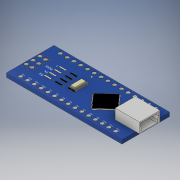
# Autodesk Inventor part: Arduino Nano
Saved by Autodesk Inventor 2019 (Build 230136000, 136)
## iProperties
Created: 2019-04-20
Part Number: Arduino Nano
Material: Generic
Document SubType Name: Modeling
Designer: richc
Density: 1 g/cm^3
Appearance: Default
Author: richc
Autodesk Inventor part; units mm, degrees
ref_plane "YZ Plane" through (0, 0, 0) normal (1, 0, 0) x (0, 1, 0)
ref_plane "XZ Plane" through (0, 0, 0) normal (0, 1, 0) x (-1, 0, 0)
ref_plane "XY Plane" through (0, 0, 0) normal (0, 0, 1) x (1, 0, 0)
sketch "Sketch1" plane through (0, 0, 0) normal (0, 1, 0) x (-1, 0, 0)
  line L0 (17.3155, -3.1926) -> (-25.8645, -3.1926)
  line L1 (-25.8645, -3.1926) -> (-25.8645, 14.5874)
  line L2 (-25.8645, 14.5874) -> (17.3155, 14.5874)
  line L3 (17.3155, 14.5874) -> (17.3155, -3.1926)
  point P0 (0, 0)
  dimension "d0" = 43.18
  dimension "d1" = 17.78
  constraints: 8 end point, 2 parallel, 1 horizontal, 1 perpendicular
  measures "d0" distance of L1.end L2.end
  measures "d1" distance of L0.end L1.end
extrude "Extrusion1" add sketch "Sketch1" along normal blind 1.524
sketch "Sketch2" plane through (0, 1.524, 0) normal (0, 1, 0) x (1, 0, 0)
  circle A0 centre (-13.5055, -13.1177) radius 0.635
  line L0 (25.8645, 3.1926) -> (-17.3155, 3.1926) projected
  line L1 (-17.3155, 3.1926) -> (-17.3155, -14.5874) projected
  line L2 (-17.3155, -14.5874) -> (25.8645, -14.5874) projected
  line L3 (25.8645, -14.5874) -> (25.8645, 3.1926) projected
  circle A1 centre (-10.9655, -13.1177) radius 0.635
  circle A2 centre (-8.4255, -13.1177) radius 0.635
  circle A3 centre (-5.8855, -13.1177) radius 0.635
  circle A4 centre (-3.3455, -13.1177) radius 0.635
  circle A5 centre (-0.8055, -13.1177) radius 0.635
  circle A6 centre (1.7345, -13.1177) radius 0.635
  circle A7 centre (4.2745, -13.1177) radius 0.635
  circle A8 centre (6.8145, -13.1177) radius 0.635
  circle A9 centre (9.3545, -13.1177) radius 0.635
  circle A10 centre (11.8945, -13.1177) radius 0.635
  circle A11 centre (14.4345, -13.1177) radius 0.635
  circle A12 centre (16.9745, -13.1177) radius 0.635
  circle A13 centre (19.5145, -13.1177) radius 0.635
  circle A14 centre (22.0545, -13.1177) radius 0.635
  line L4 (-17.3155, -5.6974) -> (-10.9655, -5.6974)
  circle A15 centre (-13.5055, 1.7229) radius 0.635
  line L5 (-17.3155, 3.1926) -> (25.8645, 3.1926)
  circle A16 centre (-10.9655, 1.7229) radius 0.635
  circle A17 centre (-8.4255, 1.7229) radius 0.635
  circle A18 centre (-5.8855, 1.7229) radius 0.635
  circle A19 centre (-3.3455, 1.7229) radius 0.635
  circle A20 centre (-0.8055, 1.7229) radius 0.635
  circle A21 centre (1.7345, 1.7229) radius 0.635
  circle A22 centre (4.2745, 1.7229) radius 0.635
  circle A23 centre (6.8145, 1.7229) radius 0.635
  circle A24 centre (9.3545, 1.7229) radius 0.635
  circle A25 centre (11.8945, 1.7229) radius 0.635
  circle A26 centre (14.4345, 1.7229) radius 0.635
  circle A27 centre (16.9745, 1.7229) radius 0.635
  circle A28 centre (19.5145, 1.7229) radius 0.635
  circle A29 centre (22.0545, 1.7229) radius 0.635
  point P0 (0, 0)
  dimension "d4" = 1.27
  dimension "d7" = 2.54
  dimension "d12" = 3.81
  constraints: 30 centre point, 15 symmetric about line, 4 end point, 2 horizontal, 1 midpoint, 43 other
  measures "d4" diameter of A0
  measures "d7" distance of A0.centre A1.centre
  measures "d12" distance from line of L1 A0.centre
extrude "Extrusion2" cut sketch "Sketch2" against normal blind 25.4 contours A0 | A1 | A2 | A3 | A4 | A5 | A6 | A7 | A8 | A9 | A10 | A11 | A12 | A13 | A14 | A15 | A16 | A17 | A18 | A19 | A20 | A21 | A22 | A23 | A24 | A25 | A26 | A27 | A28 | A29
sketch "Sketch3" plane through (0, 1.524, 0) normal (0, 1, 0) x (1, 0, 0)
  line L0 (25.8645, 3.1926) -> (-17.3155, 3.1926) projected
  line L1 (-17.3155, -14.5874) -> (25.8645, -14.5874) projected
  line L2 (10.4238, -10.3015) -> (15.5314, -5.7251)
  line L3 (15.5314, -5.7251) -> (10.9549, -0.6174)
  line L4 (5.8473, -5.1939) -> (10.9549, -0.6174)
  line L5 (5.8473, -5.1939) -> (10.4238, -10.3015)
  point P0 (0, 0)
  dimension "d26" = 6.858
  dimension "d27" = 6.858
  dimension "d28" = 6.858
  dimension "d29" = 6.858
  dimension "d75" = 90
  dimension "d76" = 3.81
  dimension "d77" = 4.2859
  constraints: 8 end point, 1 coincident
  measures "d26" distance of L4.start L2.start
  measures "d27" distance of L4.start L3.end
  measures "d28" distance of L2.end L3.end
  measures "d29" distance of L2.start L2.end
  measures "d75" angle of L2 L3
  measures "d76" distance from line of L0 L3.end
  measures "d77" distance from line of L1 L2.start
extrude "Extrusion3" add sketch "Sketch3" along normal blind 0.254
sketch "Sketch4" plane through (0, 1.524, 0) normal (0, 1, 0) x (1, 0, 0)
  circle A0 centre (-13.5055, 1.7229) radius 0.635 projected
  circle A1 centre (-13.5055, 1.7229) radius 0.7366
  line L0 (10.4238, -10.3015) -> (5.8473, -5.1939) projected
  line L1 (5.8473, -5.1939) -> (10.9549, -0.6174) projected
  line L2 (10.9549, -0.6174) -> (15.5314, -5.7251) projected
  line L3 (15.5314, -5.7251) -> (10.4238, -10.3015) projected
  circle A2 centre (-10.9655, 1.7229) radius 0.635 projected
  circle A3 centre (-5.8855, 1.7229) radius 0.635 projected
  circle A4 centre (1.7345, 1.7229) radius 0.635 projected
  circle A5 centre (22.0545, 1.7229) radius 0.635 projected
  circle A6 centre (14.4345, 1.7229) radius 0.635 projected
  circle A7 centre (9.3545, 1.7229) radius 0.635 projected
  circle A8 centre (4.2745, 1.7229) radius 0.635 projected
  circle A9 centre (22.0545, -13.1177) radius 0.635 projected
  circle A10 centre (16.9745, -13.1177) radius 0.635 projected
  circle A11 centre (11.8945, -13.1177) radius 0.635 projected
  circle A12 centre (6.8145, -13.1177) radius 0.635 projected
  circle A13 centre (1.7345, -13.1177) radius 0.635 projected
  circle A14 centre (-3.3455, -13.1177) radius 0.635 projected
  circle A15 centre (-8.4255, -13.1177) radius 0.635 projected
  circle A16 centre (-13.5055, -13.1177) radius 0.635 projected
  circle A17 centre (-10.9655, -13.1177) radius 0.635 projected
  circle A18 centre (-5.8855, -13.1177) radius 0.635 projected
  circle A19 centre (-0.8055, -13.1177) radius 0.635 projected
  circle A20 centre (4.2745, -13.1177) radius 0.635 projected
  circle A21 centre (9.3545, -13.1177) radius 0.635 projected
  circle A22 centre (14.4345, -13.1177) radius 0.635 projected
  circle A23 centre (19.5145, -13.1177) radius 0.635 projected
  circle A24 centre (-13.5055, 1.7229) radius 0.635 projected
  circle A25 centre (6.8145, 1.7229) radius 0.635 projected
  circle A26 centre (11.8945, 1.7229) radius 0.635 projected
  circle A27 centre (16.9745, 1.7229) radius 0.635 projected
  circle A28 centre (19.5145, 1.7229) radius 0.635 projected
  circle A29 centre (-3.3455, 1.7229) radius 0.635 projected
  circle A30 centre (-8.4255, 1.7229) radius 0.635 projected
  circle A31 centre (-0.8055, 1.7229) radius 0.635 projected
  line L4 (25.8645, 3.1926) -> (-17.3155, 3.1926) projected
  line L5 (-17.3155, 3.1926) -> (-17.3155, -14.5874) projected
  line L6 (-17.3155, -14.5874) -> (25.8645, -14.5874) projected
  line L7 (25.8645, -14.5874) -> (25.8645, 3.1926) projected
  circle A32 centre (-10.9655, 1.7229) radius 0.7366
  circle A33 centre (-8.4255, 1.7229) radius 0.7366
  circle A34 centre (-5.8855, 1.7229) radius 0.7366
  circle A35 centre (-3.3455, 1.7229) radius 0.7366
  circle A36 centre (-0.8055, 1.7229) radius 0.7366
  circle A37 centre (1.7345, 1.7229) radius 0.7366
  circle A38 centre (4.2745, 1.7229) radius 0.7366
  circle A39 centre (6.8145, 1.7229) radius 0.7366
  circle A40 centre (9.3545, 1.7229) radius 0.7366
  circle A41 centre (11.8945, 1.7229) radius 0.7366
  circle A42 centre (14.4345, 1.7229) radius 0.7366
  circle A43 centre (16.9745, 1.7229) radius 0.7366
  circle A44 centre (19.5145, 1.7229) radius 0.7366
  circle A45 centre (22.0545, 1.7229) radius 0.7366
  line L8 (-17.3155, 3.1926) -> (-17.3155, -14.5874) projected
  line L9 (-17.3155, -5.6974) -> (-11.7939, -5.6974)
  circle A46 centre (-13.5055, -13.1177) radius 0.635
  circle A47 centre (-13.5055, -13.1177) radius 0.7366
  circle A48 centre (-10.9655, -13.1177) radius 0.635
  circle A49 centre (-5.8855, -13.1177) radius 0.635
  circle A50 centre (1.7345, -13.1177) radius 0.635
  circle A51 centre (22.0545, -13.1177) radius 0.635
  circle A52 centre (14.4345, -13.1177) radius 0.635
  circle A53 centre (9.3545, -13.1177) radius 0.635
  circle A54 centre (4.2745, -13.1177) radius 0.635
  circle A55 centre (-13.5055, -13.1177) radius 0.635
  circle A56 centre (6.8145, -13.1177) radius 0.635
  circle A57 centre (11.8945, -13.1177) radius 0.635
  circle A58 centre (16.9745, -13.1177) radius 0.635
  circle A59 centre (19.5145, -13.1177) radius 0.635
  circle A60 centre (-3.3455, -13.1177) radius 0.635
  circle A61 centre (-8.4255, -13.1177) radius 0.635
  circle A62 centre (-0.8055, -13.1177) radius 0.635
  line L10 (25.8645, -14.5874) -> (-17.3155, -14.5874)
  line L11 (-17.3155, -14.5874) -> (-17.3155, 3.1926)
  line L12 (25.8645, 3.1926) -> (25.8645, -14.5874)
  circle A63 centre (-10.9655, -13.1177) radius 0.7366
  circle A64 centre (-8.4255, -13.1177) radius 0.7366
  circle A65 centre (-5.8855, -13.1177) radius 0.7366
  circle A66 centre (-3.3455, -13.1177) radius 0.7366
  circle A67 centre (-0.8055, -13.1177) radius 0.7366
  circle A68 centre (1.7345, -13.1177) radius 0.7366
  circle A69 centre (4.2745, -13.1177) radius 0.7366
  circle A70 centre (6.8145, -13.1177) radius 0.7366
  circle A71 centre (9.3545, -13.1177) radius 0.7366
  circle A72 centre (11.8945, -13.1177) radius 0.7366
  circle A73 centre (14.4345, -13.1177) radius 0.7366
  circle A74 centre (16.9745, -13.1177) radius 0.7366
  circle A75 centre (19.5145, -13.1177) radius 0.7366
  circle A76 centre (22.0545, -13.1177) radius 0.7366
  line L13 (-17.3155, -14.5874) -> (-17.3155, 3.1926)
  point P0 (0, 0)
  point P1 (0, -11.3949)
  dimension "d30" = 1.4732
  dimension "d33" = 2.54
  constraints: 46 centre point, 36 symmetric about line, 10 end point, 2 coincident, 2 horizontal, 1 midpoint, 59 other
  measures "d30" diameter of A1
  measures "d33" distance of A1.centre A32.centre
extrude "Extrusion4" add sketch "Sketch4" along normal blind 0.0025 contours A1 | A32 | A33 | A34 | A35 | A36 | A37 | A38 | A39 | A40 | A41 | A42 | A43 | A44 | A45 | A47 | A63 | A64 | A65 | A66 | A67 | A68 | A69 | A70 | A71 | A72 | A73 | A74 | A75 | A76
sketch "Sketch9" plane through (0, 1.524, 0) normal (0, 1, 0) x (1, 0, 0)
  line L0 (18.2445, -1.8874) -> (27.3885, -1.8874)
  line L1 (27.3885, -1.8874) -> (27.3885, -9.5074)
  line L2 (27.3885, -9.5074) -> (18.2445, -9.5074)
  line L3 (18.2445, -9.5074) -> (18.2445, -1.8874)
  line L4 (25.8645, -14.5874) -> (25.8645, 3.1926) projected
  line L5 (25.8645, -5.6974) -> (20.0043, -5.6974)
  point P0 (0, 0)
  dimension "d91" = 9.144
  dimension "d92" = 7.62
  dimension "d93" = 1.524
  constraints: 10 end point, 2 horizontal, 2 parallel, 1 midpoint, 1 perpendicular, 1 other
  measures "d91" distance of L1.end L2.end
  measures "d92" distance of L0.end L1.end
  measures "d93" distance between parallel lines of L1 L4
extrude "Extrusion5" add sketch "Sketch9" along normal blind 3.81
sketch "Sketch10" plane through (27.3885, 1.524, 9.5074) normal (1, 0, 0) x (0, 0, -1)
  line L0 (0, 0) -> (0, 3.81) projected
  line L1 (0.3159, 2.1727) -> (0.9001, 1.4006)
  line L2 (0.3159, 2.1727) -> (0.3159, 3.3797)
  line L3 (0.3159, 3.3797) -> (7.1739, 3.3797)
  line L4 (7.1739, 3.3797) -> (7.1739, 2.1727)
  line L5 (7.1739, 2.1727) -> (6.5897, 1.4006)
  line L6 (6.5897, 1.4006) -> (6.5897, 0.4656)
  line L7 (0.9001, 1.4006) -> (0.9001, 0.254)
  line L8 (-0.7941, 0.254) -> (3.7824, 0.254) projected
  line L9 (0.9001, 0.254) -> (6.5897, 0.254)
  line L10 (6.5897, 0.254) -> (6.5897, 0.4656)
  point P0 (9.5074, -1.524)
  dimension "d97" = 6.858
  dimension "d98" = 0.3159
  dimension "d125" = 0.5842
  dimension "d126" = 0.5842
  constraints: 18 end point, 3 perpendicular, 2 vertical, 1 horizontal, 1 parallel, 1 point on line
  measures "d97" distance of L4.end L1.start
  measures "d98" distance from line of L0 L1.start
  measures "d125" horizontal distance of L1.end L1.start
  measures "d126" horizontal distance of L4.end L5.end
extrude "Extrusion6" cut sketch "Sketch10" against normal blind 6.35
sketch "Sketch13" plane through (10.4238, 1.524, 10.3015) normal (-0.7447716, 0, 0.6673194) x (0.6673194, 0, 0.7447716)
  line L0 (0, 0) -> (0, 0.254) projected
  arc A0 (0, 0.207) -> (0.1323, 0.123) centre (0.1517, 0.2998) ccw
  line L1 (-15.3189, 0) -> (13.4959, 0) projected
  line L2 (0, 0.0934) -> (0.1354, 0.0303) construction
  line L3 (0, 0.0934) -> (0.1494, 0.0934) construction
  line L4 (0.1354, 0.0303) -> (0.2186, 0) construction
  line L5 (0.1354, 0.0303) -> (0.2239, 0.0303) construction
  arc A1 (0.2484, 0) -> (0.1354, 0.0303) centre (0.1697, -0.0676) ccw
  line L6 (0.1354, 0.0303) -> (0.2484, 0) construction
  line L7 (0.1354, 0.0303) -> (0.2523, 0.0303) construction
  arc A2 (0.3217, 0) -> (0.1323, 0.123) centre (0.1048, -0.1267) ccw
  line L8 (0.1323, 0.123) -> (0.3217, 0) construction
  line L9 (0.1323, 0.123) -> (0.3582, 0.123) construction
  arc A3 (0, 0.127) -> (0.1354, 0.0303) centre (0.1354, 0.1734) ccw
  line L10 (0, 0.207) -> (0, 0.127)
  line L11 (0.2484, 0) -> (0.3217, 0)
  point P0 (-14.6283, -1.524)
  dimension "d101" = 0.1778
  dimension "d103" = 25
  dimension "d105" = 20
  dimension "d106" = 15
  dimension "d107" = 33
  constraints: 20 end point, 8 point on circle, 5 point on line, 4 centre point, 4 equal length, 4 horizontal, 2 tangent, 1 collinear, 1 midpoint, 1 vertical
  measures "d101" radius of A0
  measures "d103" angle of L2 L3
  measures "d105" angle of L4 L5
  measures "d106" angle of L6 L7
  measures "d107" angle of L8 L9
extrude "Extrusion7" add sketch "Sketch13" against normal blind 6.858 contours L0 A0 A2 L1 A1 A3
sketch "Sketch14" plane through (5.8473, 1.524, 5.1939) normal (-0.6673194, 0, -0.7447716) x (-0.7447716, 0, 0.6673194)
  line L0 (0, 0) -> (0, 0.254)
  arc A0 (0, 0.207) -> (0.1323, 0.123) centre (0.1517, 0.2998) ccw
  line L1 (-15.3189, 0) -> (13.4959, 0)
  line L2 (0, 0.0934) -> (0.1354, 0.0303) construction
  line L3 (0, 0.0934) -> (0.1494, 0.0934) construction
  line L4 (0.1354, 0.0303) -> (0.2186, 0) construction
  line L5 (0.1354, 0.0303) -> (0.2239, 0.0303) construction
  arc A1 (0.2484, 0) -> (0.1354, 0.0303) centre (0.1697, -0.0676) ccw
  line L6 (0.1354, 0.0303) -> (0.2484, 0) construction
  line L7 (0.1354, 0.0303) -> (0.2523, 0.0303) construction
  arc A2 (0.3217, 0) -> (0.1323, 0.123) centre (0.1048, -0.1267) ccw
  line L8 (0.1323, 0.123) -> (0.3217, 0) construction
  line L9 (0.1323, 0.123) -> (0.3582, 0.123) construction
  arc A3 (0, 0.127) -> (0.1354, 0.0303) centre (0.1354, 0.1734) ccw
  line L10 (0, 0.207) -> (0, 0.127)
  line L11 (0.2484, 0) -> (0.3217, 0)
  point P0 (0.8889, -1.524)
  dimension "d110" = 0.1778
  dimension "d111" = 25
  dimension "d112" = 20
  dimension "d113" = 15
  dimension "d114" = 33
  constraints: 24 end point, 8 point on circle, 5 point on line, 4 centre point, 4 equal length, 4 horizontal, 2 tangent, 1 collinear, 1 midpoint, 1 vertical
  measures "d110" radius of A0
  measures "d111" angle of L2 L3
  measures "d112" angle of L4 L5
  measures "d113" angle of L6 L7
  measures "d114" angle of L8 L9
extrude "Extrusion8" add sketch "Sketch14" against normal blind 6.858 contours L0 A0 A2 L1 A1 A3
sketch "Sketch15" plane through (10.9549, 1.524, 0.6174) normal (0.7447716, 0, -0.6673194) x (-0.6673194, 0, -0.7447716)
  line L0 (0, 0) -> (0, 0.254)
  arc A0 (0, 0.207) -> (0.1323, 0.123) centre (0.1517, 0.2998) ccw
  line L1 (-15.3189, 0) -> (13.4959, 0)
  line L2 (0, 0.0934) -> (0.1354, 0.0303) construction
  line L3 (0, 0.0934) -> (0.1494, 0.0934) construction
  line L4 (0.1354, 0.0303) -> (0.2186, 0) construction
  line L5 (0.1354, 0.0303) -> (0.2239, 0.0303) construction
  arc A1 (0.2484, 0) -> (0.1354, 0.0303) centre (0.1697, -0.0676) ccw
  line L6 (0.1354, 0.0303) -> (0.2484, 0) construction
  line L7 (0.1354, 0.0303) -> (0.2523, 0.0303) construction
  arc A2 (0.3217, 0) -> (0.1323, 0.123) centre (0.1048, -0.1267) ccw
  line L8 (0.1323, 0.123) -> (0.3217, 0) construction
  line L9 (0.1323, 0.123) -> (0.3582, 0.123) construction
  arc A3 (0, 0.127) -> (0.1354, 0.0303) centre (0.1354, 0.1734) ccw
  line L10 (0, 0.207) -> (0, 0.127)
  line L11 (0.2484, 0) -> (0.3217, 0)
  point P0 (7.7703, -1.524)
  dimension "d117" = 0.1778
  dimension "d118" = 25
  dimension "d119" = 20
  dimension "d120" = 15
  dimension "d121" = 33
  constraints: 24 end point, 8 point on circle, 5 point on line, 4 centre point, 4 equal length, 4 horizontal, 2 tangent, 1 collinear, 1 midpoint, 1 vertical
  measures "d117" radius of A0
  measures "d118" angle of L2 L3
  measures "d119" angle of L4 L5
  measures "d120" angle of L6 L7
  measures "d121" angle of L8 L9
extrude "Extrusion9" add sketch "Sketch15" against normal blind 6.858 contours L0 A0 A2 L1 A1 A3
sketch "Sketch19" plane through (10.9549, 1.778, 0.6174) normal (-0.6673194, 0, -0.7447716) x (-0.7447716, 0, 0.6673194)
  line L0 (0, 0) -> (0, 0.254)
  arc A0 (0, 0.207) -> (0.1323, 0.123) centre (0.1517, 0.2998) ccw
  line L1 (-15.3189, 0) -> (13.4959, 0)
  line L2 (0, 0.0934) -> (0.1354, 0.0303) construction
  line L3 (0, 0.0934) -> (0.1494, 0.0934) construction
  line L4 (0.1354, 0.0303) -> (0.2186, 0) construction
  line L5 (0.1354, 0.0303) -> (0.2239, 0.0303) construction
  arc A1 (0.2484, 0) -> (0.1354, 0.0303) centre (0.1697, -0.0676) ccw
  line L6 (0.1354, 0.0303) -> (0.2484, 0) construction
  line L7 (0.1354, 0.0303) -> (0.2523, 0.0303) construction
  arc A2 (0.3217, 0) -> (0.1323, 0.123) centre (0.1048, -0.1267) ccw
  line L8 (0.1323, 0.123) -> (0.3217, 0) construction
  line L9 (0.1323, 0.123) -> (0.3582, 0.123) construction
  arc A3 (0, 0.127) -> (0.1354, 0.0303) centre (0.1354, 0.1734) ccw
  line L10 (0, 0.207) -> (0, 0.127)
  line L11 (0.2484, 0) -> (0.3217, 0)
  line L12 (0, -0.1606) -> (-0.1494, -0.1606) construction
  arc A4 (-0.1354, -0.2237) -> (0, -0.127) centre (-0.1354, -0.0806) ccw
  line L13 (0, -0.1606) -> (-0.1354, -0.2237) construction
  arc A5 (-0.1323, -0.131) -> (0, -0.047) centre (-0.1517, 0.0458) ccw
  line L14 (-0.1354, -0.2237) -> (-0.2239, -0.2237) construction
  arc A6 (-0.1354, -0.2237) -> (-0.2484, -0.254) centre (-0.1697, -0.3216) ccw
  line L15 (-0.1354, -0.2237) -> (-0.2523, -0.2237) construction
  line L16 (-0.1323, -0.131) -> (-0.3217, -0.254) construction
  arc A7 (-0.1323, -0.131) -> (-0.3217, -0.254) centre (-0.1048, -0.3807) ccw
  line L17 (-0.1323, -0.131) -> (-0.3582, -0.131) construction
  line L18 (0, -0.131) -> (0, -0.047) projected
  line L19 (0, -0.131) -> (6.858, -0.131) projected
  line L20 (6.858, -0.047) -> (6.858, -0.131) projected
  line L21 (0, -0.047) -> (6.858, -0.047) projected
  line L22 (-0.3217, -0.254) -> (-0.2484, -0.254)
  line L23 (-1.1064, -0.254) -> (0.3668, -0.254) projected
  line L24 (6.858, -0.127) -> (0, -0.127) projected
  line L25 (0, -0.047) -> (0, -0.127)
  point P0 (7.7469, -1.778)
  dimension "d127" = 0.1778
  dimension "d128" = 25
  dimension "d129" = 20
  dimension "d130" = 15
  dimension "d131" = 33
  constraints: 40 end point, 18 point on circle, 8 centre point, 5 point on line, 4 equal length, 4 horizontal, 2 collinear, 2 tangent, 1 vertical
  measures "d127" radius of A0
  measures "d128" angle of L2 L3
  measures "d129" angle of L4 L5
  measures "d130" angle of L6 L7
  measures "d131" angle of L8 L9
extrude "Extrusion10" add sketch "Sketch19" against normal blind 6.858 contours A6 L22 A7 A5 L18 A4
sketch "Sketch20" plane through (0, 1.524, 0) normal (0, 1, 0) x (1, 0, 0)
  line L0 (-17.3155, 3.1926) -> (-17.3155, -14.5874) projected
  line L1 (-17.3155, -1.3474) -> (-17.3155, -9.7681)
  circle A0 centre (-16.4061, -8.1104) radius 0.635
  circle A1 centre (-14.3158, -8.1104) radius 0.635
  circle A2 centre (-16.4061, -5.5704) radius 0.635
  circle A3 centre (-14.3158, -5.5704) radius 0.635
  circle A4 centre (-16.4061, -3.0304) radius 0.635
  circle A5 centre (-14.3158, -3.0304) radius 0.635
  line L2 (-17.3155, -8.9994) -> (-13.4268, -8.9994)
  line L3 (-13.4268, -8.9994) -> (-13.4268, -2.1414)
  line L4 (-13.4268, -2.1414) -> (-17.3155, -2.1414)
  line L5 (-17.3155, -2.1414) -> (-17.3155, -8.9994)
  line L6 (25.8645, 3.1926) -> (-17.3155, 3.1926) projected
  point P0 (0, 0)
  dimension "d134" = 1.27
  dimension "d135" = 1.27
  dimension "d138" = 2.54
  dimension "d144" = 11.303
  dimension "d145" = 11.303
  dimension "d146" = 0.889
  dimension "d147" = 0.889
  dimension "d148" = 0.889
  constraints: 10 end point, 6 centre point, 2 parallel, 2 point on line, 1 horizontal, 1 perpendicular, 1 vertical, 8 other
  measures "d134" diameter of A0
  measures "d135" diameter of A1
  measures "d138" distance of A0.centre A2.centre
  measures "d144" distance from line of L6 A0.centre
  measures "d145" distance from line of L6 A1.centre
  measures "d146" distance from line of A0.centre L2
  measures "d147" distance from line of L4 A4.centre
  measures "d148" distance from line of L3 A1.centre
extrude "Extrusion11" cut sketch "Sketch20" against normal blind 6.858 contours A0 | A1 | A2 | A3 | A4 | A5
sketch "Sketch21" plane through (0, 1.524, 0) normal (0, 1, 0) x (1, 0, 0)
  circle A0 centre (-16.4061, -3.0304) radius 0.635 projected
  circle A1 centre (-16.4061, -5.5704) radius 0.635 projected
  circle A2 centre (-16.4061, -8.1104) radius 0.635 projected
  circle A3 centre (-14.3158, -8.1104) radius 0.635 projected
  circle A4 centre (-14.3158, -5.5704) radius 0.635 projected
  circle A5 centre (-14.3158, -3.0304) radius 0.635 projected
  line L0 (15.7164, -5.5593) -> (11.1399, -0.4517) projected
  line L1 (11.1399, -0.4517) -> (11.1945, -0.4027) projected
  line L2 (11.1945, -0.4027) -> (15.771, -5.5104) projected
  line L3 (15.771, -5.5104) -> (15.7164, -5.5593) projected
  line L4 (10.7892, -0.4325) -> (5.6816, -5.0089) projected
  line L5 (5.6816, -5.0089) -> (5.6326, -4.9543) projected
  line L6 (5.6326, -4.9543) -> (10.7403, -0.3778) projected
  line L7 (10.7403, -0.3778) -> (10.7892, -0.4325) projected
  line L8 (5.6623, -5.3596) -> (10.2388, -10.4673) projected
  line L9 (10.2388, -10.4673) -> (10.1842, -10.5162) projected
  line L10 (10.1842, -10.5162) -> (5.6077, -5.4086) projected
  line L11 (5.6077, -5.4086) -> (5.6623, -5.3596) projected
  line L12 (15.7461, -5.9647) -> (10.6385, -10.5412) projected
  line L13 (10.6385, -10.5412) -> (10.5895, -10.4865) projected
  line L14 (10.5895, -10.4865) -> (15.6971, -5.91) projected
  line L15 (15.6971, -5.91) -> (15.7461, -5.9647) projected
  line L16 (18.2445, -1.8874) -> (25.8645, -1.8874) projected
  line L17 (25.8645, -1.8874) -> (25.8645, 3.1926) projected
  line L18 (25.8645, 3.1926) -> (-17.3155, 3.1926) projected
  line L19 (-17.3155, 3.1926) -> (-17.3155, -14.5874) projected
  line L20 (-17.3155, -14.5874) -> (25.8645, -14.5874) projected
  line L21 (25.8645, -14.5874) -> (25.8645, -9.5074) projected
  line L22 (25.8645, -9.5074) -> (18.2445, -9.5074) projected
  line L23 (18.2445, -9.5074) -> (18.2445, -1.8874) projected
  circle A6 centre (-8.4255, -13.1177) radius 0.7366 projected
  circle A7 centre (-3.3455, -13.1177) radius 0.7366 projected
  circle A8 centre (-0.8055, -13.1177) radius 0.7366 projected
  circle A9 centre (6.8145, -13.1177) radius 0.7366 projected
  circle A10 centre (9.3545, -13.1177) radius 0.7366 projected
  circle A11 centre (16.9745, -13.1177) radius 0.7366 projected
  circle A12 centre (11.8945, -13.1177) radius 0.7366 projected
  circle A13 centre (22.0545, 1.7229) radius 0.7366 projected
  circle A14 centre (16.9745, 1.7229) radius 0.7366 projected
  circle A15 centre (11.8945, 1.7229) radius 0.7366 projected
  circle A16 centre (6.8145, 1.7229) radius 0.7366 projected
  circle A17 centre (1.7345, 1.7229) radius 0.7366 projected
  circle A18 centre (-3.3455, 1.7229) radius 0.7366 projected
  circle A19 centre (-8.4255, 1.7229) radius 0.7366 projected
  circle A20 centre (-13.5055, 1.7229) radius 0.7366 projected
  circle A21 centre (-10.9655, 1.7229) radius 0.7366 projected
  circle A22 centre (-5.8855, 1.7229) radius 0.7366 projected
  circle A23 centre (-0.8055, 1.7229) radius 0.7366 projected
  circle A24 centre (4.2745, 1.7229) radius 0.7366 projected
  circle A25 centre (9.3545, 1.7229) radius 0.7366 projected
  circle A26 centre (14.4345, 1.7229) radius 0.7366 projected
  circle A27 centre (19.5145, 1.7229) radius 0.7366 projected
  circle A28 centre (14.4345, -13.1177) radius 0.7366 projected
  circle A29 centre (-13.5055, -13.1177) radius 0.7366 projected
  circle A30 centre (19.5145, -13.1177) radius 0.7366 projected
  circle A31 centre (4.2745, -13.1177) radius 0.7366 projected
  circle A32 centre (22.0545, -13.1177) radius 0.7366 projected
  circle A33 centre (1.7345, -13.1177) radius 0.7366 projected
  circle A34 centre (-5.8855, -13.1177) radius 0.7366 projected
  circle A35 centre (-10.9655, -13.1177) radius 0.7366 projected
  line L24 (10.4238, -10.3015) -> (5.8473, -5.1939) projected
  line L25 (5.8473, -5.1939) -> (10.9549, -0.6174) projected
  line L26 (10.9549, -0.6174) -> (15.5314, -5.7251) projected
  line L27 (15.5314, -5.7251) -> (10.4238, -10.3015) projected
  circle A36 centre (-16.4061, -3.0304) radius 0.7366
  circle A37 centre (-14.3158, -3.0304) radius 0.7366
  circle A38 centre (-14.3158, -5.5704) radius 0.7366
  circle A39 centre (-16.4061, -5.5704) radius 0.7366
  circle A40 centre (-16.4061, -8.1104) radius 0.7366
  circle A41 centre (-14.3158, -8.1104) radius 0.7366
  point P0 (0, 0)
  dimension "d151" = 1.4732
  dimension "d152" = 1.4732
  dimension "d153" = 1.4732
  dimension "d154" = 1.4732
  dimension "d155" = 1.4732
  dimension "d156" = 1.4732
  constraints: 6 centre point, 6 coincident
  measures "d151" diameter of A36
  measures "d152" diameter of A37
  measures "d153" diameter of A38
  measures "d154" diameter of A39
  measures "d155" diameter of A40
  measures "d156" diameter of A41
extrude "Extrusion12" add sketch "Sketch21" along normal blind 0.0025 contours A36 | A37 | A38 | A39 | A40 | A41
sketch "Sketch22" plane through (0, 1.524, 0) normal (0, 1, 0) x (1, 0, 0)
  line L0 (1.7757, -3.0304) -> (-0.7643, -3.0304)
  line L1 (-0.7643, -3.0304) -> (-0.7643, -8.1104)
  line L2 (-0.7643, -8.1104) -> (1.7757, -8.1104)
  line L3 (1.7757, -8.1104) -> (1.7757, -3.0304)
  point P0 (0, 0)
  dimension "d159" = 5.08
  dimension "d160" = 2.54
  constraints: 8 end point, 2 parallel, 1 horizontal, 1 perpendicular
  measures "d159" distance of L2.end L0.start
  measures "d160" distance of L0.start L0.end
extrude "Extrusion13" add sketch "Sketch22" along normal blind 0.508
sketch "Sketch23" plane through (0, 2.032, 0) normal (0, 1, 0) x (1, 0, 0)
  line L0 (-0.5611, -3.2336) -> (1.5725, -3.2336)
  line L1 (1.5725, -3.2336) -> (1.5725, -7.9072)
  line L2 (1.5725, -7.9072) -> (-0.5611, -7.9072)
  line L3 (-0.5611, -7.9072) -> (-0.5611, -3.2336)
  line L4 (1.7757, -8.1104) -> (1.7757, -3.0304) projected
  line L5 (-0.7643, -3.0304) -> (-0.7643, -8.1104) projected
  line L6 (1.7757, -3.0304) -> (-0.7643, -3.0304) projected
  line L7 (-0.7643, -8.1104) -> (1.7757, -8.1104) projected
  point P0 (0, 0)
  dimension "d163" = 0.2032
  dimension "d164" = 0.2032
  dimension "d165" = 0.2032
  dimension "d166" = 0.2032
  constraints: 8 end point, 2 parallel, 1 horizontal, 1 perpendicular
  measures "d163" distance between parallel lines of L4 L1
  measures "d164" distance between parallel lines of L5 L3
  measures "d165" distance between parallel lines of L6 L0
  measures "d166" distance between parallel lines of L7 L2
extrude "Extrusion14" add sketch "Sketch23" along normal blind 0.1778 contours L0 L1 L2 L3
sketch "Sketch24" plane through (0, 2.2098, 0) normal (0, 1, 0) x (1, 0, 0)
  line L0 (-0.2817, -3.513) -> (1.2931, -3.513)
  line L1 (1.2931, -3.513) -> (1.2931, -7.6278)
  line L2 (1.2931, -7.6278) -> (-0.2817, -7.6278)
  line L3 (-0.2817, -7.6278) -> (-0.2817, -3.513)
  line L4 (1.5725, -3.2336) -> (-0.5611, -3.2336) projected
  line L5 (-0.5611, -7.9072) -> (1.5725, -7.9072) projected
  line L6 (1.5725, -7.9072) -> (1.5725, -3.2336) projected
  line L7 (-0.5611, -3.2336) -> (-0.5611, -7.9072) projected
  point P0 (0, 0)
  dimension "d169" = 0.2794
  dimension "d170" = 0.2794
  dimension "d171" = 0.2794
  dimension "d172" = 0.2794
  constraints: 8 end point, 2 parallel, 1 horizontal, 1 perpendicular
  measures "d169" distance between parallel lines of L4 L0
  measures "d170" distance between parallel lines of L5 L2
  measures "d171" distance between parallel lines of L6 L1
  measures "d172" distance between parallel lines of L7 L3
extrude "Extrusion15" add sketch "Sketch24" along normal blind 0.381 contours L0 L1 L2 L3
fillet "Fillet1" radius 0.0762 4 edges at (1.2931, 2.4003, 7.6278) (-0.2817, 2.4003, 7.6278) (1.2931, 2.4003, 3.513) (-0.2817, 2.4003, 3.513)
sketch "Sketch25" plane through (1.7757, 1.524, 8.1104) normal (1, 0, 0) x (0, 0, -1)
  line L0 (0.1354, 0.0303) -> (0.2186, 0) construction
  line L1 (0.1354, 0.0303) -> (0.2239, 0.0303) construction
  line L2 (0.1354, 0.0303) -> (0.2484, 0) construction
  line L3 (0.1354, 0.0303) -> (0.2523, 0.0303) construction
  line L4 (0.2484, 0) -> (0.3217, 0)
  arc A0 (0.2484, 0) -> (0.1354, 0.0303) centre (0.1697, -0.0676) ccw
  line L5 (0.1323, 0.123) -> (0.3217, 0) construction
  line L6 (0.1323, 0.123) -> (0.3582, 0.123) construction
  arc A1 (0.3217, 0) -> (0.1323, 0.123) centre (0.1048, -0.1267) ccw
  line L7 (0, 0.0934) -> (0.1354, 0.0303) construction
  line L8 (0, 0.0934) -> (0.1494, 0.0934) construction
  arc A2 (0, 0.127) -> (0.1354, 0.0303) centre (0.1354, 0.1734) ccw
  line L9 (0, 0.207) -> (0, 0.127)
  arc A3 (0, 0.207) -> (0.1323, 0.123) centre (0.1517, 0.2998) ccw
  line L10 (0, 0) -> (0, 0.254)
  line L11 (-15.3189, 0) -> (13.4959, 0)
  line L12 (-0.1354, 0.0303) -> (-0.2186, 0) construction
  line L13 (-0.1354, 0.0303) -> (-0.2239, 0.0303) construction
  line L14 (-0.1354, 0.0303) -> (-0.2484, 0) construction
  line L15 (-0.1354, 0.0303) -> (-0.2523, 0.0303) construction
  line L16 (-0.1323, 0.123) -> (-0.3217, 0) construction
  line L17 (-0.1323, 0.123) -> (-0.3582, 0.123) construction
  arc A4 (-0.1354, 0.0303) -> (-0.2484, 0) centre (-0.1697, -0.0676) ccw
  arc A5 (-0.1323, 0.123) -> (-0.3217, 0) centre (-0.1048, -0.1267) ccw
  arc A6 (-0.1323, 0.123) -> (0, 0.207) centre (-0.1517, 0.2998) ccw
  arc A7 (-0.1354, 0.0303) -> (0, 0.127) centre (-0.1354, 0.1734) ccw
  line L18 (0, 0.0934) -> (-0.1354, 0.0303) construction
  line L19 (0, 0.0934) -> (-0.1494, 0.0934) construction
  line L20 (-0.3217, 0) -> (-0.2484, 0)
  line L21 (0, 0.207) -> (0, 0.127)
  line L22 (0, 0) -> (0, 0.508) projected
  point P0 (8.1104, -1.524)
  dimension "d176" = 0.1778
  dimension "d177" = 25
  dimension "d178" = 20
  dimension "d179" = 15
  dimension "d180" = 33
  constraints: 44 end point, 16 point on circle, 13 symmetric about line, 8 centre point, 5 point on line, 4 equal length, 4 horizontal, 3 collinear, 2 tangent, 1 midpoint, 1 vertical, 4 other
  measures "d176" radius of A3
  measures "d177" angle of L7 L8
  measures "d178" angle of L0 L1
  measures "d179" angle of L2 L3
  measures "d180" angle of L5 L6
extrude "Extrusion16" add sketch "Sketch25" against normal blind 2.286 contours A7 A4 L11 A5 A6 L9
sketch "Sketch27" plane through (-0.7643, 1.524, 3.0304) normal (-1, 0, 0) x (0, 0, 1)
  line L0 (-0.1354, 0.0303) -> (-0.2239, 0.0303) construction
  line L1 (-0.1354, 0.0303) -> (-0.2484, 0) construction
  arc A0 (-0.1354, 0.0303) -> (-0.2484, 0) centre (-0.1697, -0.0676) ccw
  line L2 (-0.1354, 0.0303) -> (-0.2523, 0.0303) construction
  line L3 (-0.1323, 0.123) -> (-0.3217, 0) construction
  arc A1 (-0.1323, 0.123) -> (-0.3217, 0) centre (-0.1048, -0.1267) ccw
  line L4 (0, 0.0934) -> (-0.1354, 0.0303) construction
  arc A2 (-0.1354, 0.0303) -> (0, 0.127) centre (-0.1354, 0.1734) ccw
  line L5 (-0.1323, 0.123) -> (-0.3582, 0.123) construction
  arc A3 (-0.1323, 0.123) -> (0, 0.207) centre (-0.1517, 0.2998) ccw
  line L6 (0, 0.0934) -> (-0.1494, 0.0934) construction
  line L7 (-0.1354, 0.0303) -> (-0.2186, 0) construction
  line L8 (-0.3217, 0) -> (-0.2389, 0.0025)
  line L9 (-0.635, 0.0025) -> (0.635, 0.0025) projected
  line L10 (0, 0.127) -> (0, 0.207)
  line L11 (0, 0) -> (0, 0.508) projected
  line L12 (-0.3217, 0) -> (-0.2484, 0)
  point P0 (-3.0304, -1.524)
  constraints: 22 end point, 8 point on circle, 4 centre point, 2 point on line, 1 collinear, 1 parallel
extrude "Extrusion17" add sketch "Sketch27" against normal blind 2.286 contours A0 L9 A1 A3 L10 A2 | A0 L12 L8 | L8 A1 L9
sketch "Sketch28" plane through (0, 2.032, 0) normal (0, 1, 0) x (1, 0, 0)
  line L0 (-0.5103, -8.1104) -> (-0.5103, -8.2459) projected
  line L1 (-0.5103, -8.1104) -> (0.2347, -8.1104)
  line L2 (0.2347, -8.1104) -> (0.2347, -8.4385)
  line L3 (0.2347, -8.4385) -> (-0.5103, -8.4385)
  line L4 (-0.5103, -8.4385) -> (-0.5103, -8.1104)
  line L5 (1.7757, -8.1104) -> (-0.7643, -8.1104) projected
  line L6 (1.7757, -8.3588) -> (1.7757, -8.4321) projected
  line L7 (0.7768, -8.1104) -> (1.7757, -8.1104)
  line L8 (1.7757, -8.1104) -> (1.7757, -8.4321)
  line L9 (1.7757, -8.4321) -> (0.7768, -8.4321)
  line L10 (0.7768, -8.4321) -> (0.7768, -8.1104)
  line L11 (1.2169, -7.6278) -> (-0.2055, -7.6278) projected
  line L12 (0.5057, -7.6278) -> (0.5057, -8.0013)
  line L13 (1.7757, -8.4321) -> (-0.5103, -8.4321) projected
  line L14 (0.2347, -8.1104) -> (0.4273, -8.1104)
  line L15 (0.4273, -8.1104) -> (0.4273, -8.4321)
  line L16 (0.4273, -8.4321) -> (0.2347, -8.4321)
  line L17 (0.2347, -8.4321) -> (0.2347, -8.1104)
  line L18 (0.7768, -8.1104) -> (0.5842, -8.1104)
  line L19 (0.5842, -8.1104) -> (0.5842, -8.4321)
  line L20 (0.5842, -8.4321) -> (0.7768, -8.4321)
  line L21 (0.7768, -8.4321) -> (0.7768, -8.1104)
  line L22 (1.2931, -7.5516) -> (1.2931, -3.5892) projected
  line L23 (1.2931, -5.5704) -> (0.6805, -5.5704)
  line L24 (-0.5103, -3.0304) -> (-0.5103, -2.895)
  line L25 (-0.5103, -3.0304) -> (0.2347, -3.0304)
  line L26 (0.2347, -3.0304) -> (0.2347, -2.7023)
  line L27 (0.2347, -2.7023) -> (-0.5103, -2.7023)
  line L28 (-0.5103, -2.7023) -> (-0.5103, -3.0304)
  line L29 (1.7757, -3.0304) -> (-0.7643, -3.0304)
  line L30 (1.7757, -2.7821) -> (1.7757, -2.7087)
  line L31 (0.7768, -3.0304) -> (1.7757, -3.0304)
  line L32 (1.7757, -3.0304) -> (1.7757, -2.7087)
  line L33 (1.7757, -2.7087) -> (0.7768, -2.7087)
  line L34 (0.7768, -2.7087) -> (0.7768, -3.0304)
  line L35 (1.7757, -2.7087) -> (-0.5103, -2.7087)
  line L36 (0.2347, -3.0304) -> (0.4273, -3.0304)
  line L37 (0.4273, -3.0304) -> (0.4273, -2.7087)
  line L38 (0.4273, -2.7087) -> (0.2347, -2.7087)
  line L39 (0.2347, -2.7087) -> (0.2347, -3.0304)
  line L40 (0.7768, -3.0304) -> (0.5842, -3.0304)
  line L41 (0.5842, -3.0304) -> (0.5842, -2.7087)
  line L42 (0.5842, -2.7087) -> (0.7768, -2.7087)
  line L43 (0.7768, -2.7087) -> (0.7768, -3.0304)
  line L44 (-0.7643, -2.7821) -> (-0.7643, -2.7087) projected
  line L45 (-0.7643, -2.7087) -> (-0.5103, -2.7087)
  line L46 (-0.5103, -2.7087) -> (-0.5103, -3.0304)
  line L47 (-0.5103, -3.0304) -> (-0.7643, -3.0304)
  line L48 (-0.7643, -3.0304) -> (-0.7643, -2.7087)
  point P0 (0, 0)
  constraints: 84 end point, 19 symmetric about line, 10 parallel, 6 horizontal, 6 point on line, 5 perpendicular, 2 midpoint, 1 vertical, 2 other
extrude "Extrusion18" cut sketch "Sketch28" against normal blind 0.508 contours L1 L2 L13 L4 L0 | L5 L15 L13 L2 | L13 L2 L3 L4 | L5 L10 L13 L19 | L5 L8 L6 L9 L10 | L29 L48 L44 L45 L28 L24 | L24 L28 L35 L26 L25 | L26 L35 L37 L29 | L28 L27 L26 L35 | L41 L35 L34 L29 | L34 L33 L30 L32 L29
sketch "Sketch30" plane through (0, 1.524, 0) normal (0, 1, 0) x (1, 0, 0)
  line L0 (-17.3155, -14.5874) -> (-17.3155, 3.1926) projected
  line L1 (-17.3155, -1.8874) -> (-13.3785, -1.8874)
  line L2 (-13.3785, -1.8874) -> (-13.3785, -9.2534)
  line L3 (-13.3785, -9.2534) -> (-17.3155, -9.2534)
  line L4 (-17.3155, -9.2534) -> (-17.3155, -1.8874)
  line L5 (25.8645, 3.1926) -> (-17.3155, 3.1926) projected
  line L6 (-17.3155, -1.7604) -> (-13.2515, -1.7604)
  line L7 (-13.2515, -1.7604) -> (-13.2515, -9.3804)
  line L8 (-13.2515, -9.3804) -> (-17.3155, -9.3804)
  line L9 (-17.3155, -9.3804) -> (-17.3155, -1.7604)
  point P0 (0, 0)
  dimension "d187" = 7.366
  dimension "d188" = 5.08
  dimension "d189" = 3.937
  dimension "d191" = 4.064
  dimension "d192" = 0.127
  dimension "d193" = 0.127
  constraints: 16 end point, 4 parallel, 2 horizontal, 2 perpendicular, 2 point on line
  measures "d187" distance between parallel lines of L3 L1
  measures "d188" distance between parallel lines of L5 L1
  measures "d189" distance of L1.start L1.end
  measures "d191" distance of L6.start L6.end
  measures "d192" distance between parallel lines of L3 L8
  measures "d193" distance between parallel lines of L6 L1
extrude "Extrusion19" add sketch "Sketch30" along normal blind 0.0003 contours L0 L3 L2 L1 L6 L7 L8
sketch "Sketch31" plane through (0, 1.524, 0) normal (0, 1, 0) x (1, 0, 0)
  line L0 (-2.7477, -3.0304) -> (-5.2877, -3.0304)
  line L1 (-5.2877, -3.0304) -> (-5.2877, -2.5224)
  line L2 (-5.2877, -2.5224) -> (-2.7477, -2.5224)
  line L3 (-2.7477, -2.5224) -> (-2.7477, -3.0304)
  line L4 (-0.7643, -3.0304) -> (1.7757, -3.0304) projected
  line L5 (-0.7643, -3.0304) -> (-13.3069, -3.0304)
  line L6 (1.7757, -8.1104) -> (-0.7643, -8.1104) projected
  line L7 (-9.3517, -3.0304) -> (-6.8117, -3.0304)
  line L8 (-6.8117, -3.0304) -> (-6.8117, -2.5224)
  line L9 (-6.8117, -2.5224) -> (-9.3517, -2.5224)
  line L10 (-9.3517, -2.5224) -> (-9.3517, -3.0304)
  line L11 (-0.7643, -3.0304) -> (-0.7643, -8.1104) projected
  line L12 (-0.5611, -3.2336) -> (-0.5611, -7.9072) projected
  line L13 (-2.7477, -4.3851) -> (-2.7477, -4.8931)
  line L14 (-2.7477, -4.8931) -> (-5.2877, -4.8931)
  line L15 (-5.2877, -4.8931) -> (-5.2877, -4.3851)
  line L16 (-5.2877, -4.3851) -> (-2.7477, -4.3851)
  line L17 (-6.8117, -4.8931) -> (-6.8117, -4.3851)
  line L18 (-9.3517, -4.8931) -> (-6.8117, -4.8931)
  line L19 (-6.8117, -4.3851) -> (-9.3517, -4.3851)
  line L20 (-9.3517, -4.3851) -> (-9.3517, -4.8931)
  line L21 (-0.7643, -4.8931) -> (-13.3069, -4.8931)
  line L22 (-2.7477, -6.2477) -> (-2.7477, -6.7557)
  line L23 (-2.7477, -6.7557) -> (-5.2877, -6.7557)
  line L24 (-5.2877, -6.7557) -> (-5.2877, -6.2477)
  line L25 (-5.2877, -6.2477) -> (-2.7477, -6.2477)
  line L26 (-6.8117, -6.7557) -> (-6.8117, -6.2477)
  line L27 (-9.3517, -6.7557) -> (-6.8117, -6.7557)
  line L28 (-6.8117, -6.2477) -> (-9.3517, -6.2477)
  line L29 (-9.3517, -6.2477) -> (-9.3517, -6.7557)
  line L30 (-0.7643, -6.7557) -> (-13.3069, -6.7557)
  line L31 (-2.7477, -8.1104) -> (-2.7477, -8.6184)
  line L32 (-2.7477, -8.6184) -> (-5.2877, -8.6184)
  line L33 (-5.2877, -8.6184) -> (-5.2877, -8.1104)
  line L34 (-5.2877, -8.1104) -> (-2.7477, -8.1104)
  line L35 (-6.8117, -8.6184) -> (-6.8117, -8.1104)
  line L36 (-9.3517, -8.6184) -> (-6.8117, -8.6184)
  line L37 (-6.8117, -8.1104) -> (-9.3517, -8.1104)
  line L38 (-9.3517, -8.1104) -> (-9.3517, -8.6184)
  line L39 (-0.7643, -8.6184) -> (-13.3069, -8.6184)
  line L40 (0.4273, -2.8982) -> (0.4273, -2.7087) projected
  point P0 (0, 0)
  dimension "d196" = 2.54
  dimension "d197" = 0.508
  dimension "d198" = 2.54
  dimension "d199" = 0.508
  dimension "d202" = 1.8627
  dimension "d207" = 3.175
  dimension "d208" = 1.524
  constraints: 72 end point, 8 point on line, 4 parallel, 3 horizontal, 2 perpendicular, 1 vertical, 57 other
  measures "d196" distance of L1.end L2.end
  measures "d197" distance of L2.end L0.start
  measures "d198" distance of L9.end L8.end
  measures "d199" distance of L8.end L7.end
  measures "d202" distance of L0.start L13.end
  measures "d207" distance between parallel lines of L40 L3
  measures "d208" distance between parallel lines of L1 L8
extrude "Extrusion20" add sketch "Sketch31" along normal blind 0.127
sketch "Sketch32" plane through (0, 1.524, 0) normal (0, 1, 0) x (1, 0, 0)
  line L0 (-9.3872, -2.5123) -> (-6.7761, -2.5123)
  line L1 (-6.7761, -2.5123) -> (-6.7761, -3.0406)
  line L2 (-6.7761, -3.0406) -> (-9.3872, -3.0406)
  line L3 (-9.3872, -3.0406) -> (-9.3872, -2.5123)
  line L4 (-6.8117, -2.5224) -> (-9.3517, -2.5224) projected
  line L5 (-9.3517, -3.0304) -> (-6.8117, -3.0304) projected
  line L6 (-6.8117, -3.0304) -> (-6.8117, -2.5224) projected
  line L7 (-9.3517, -2.5224) -> (-9.3517, -3.0304) projected
  line L8 (-2.7477, -2.5224) -> (-5.2877, -2.5224) projected
  line L9 (-6.8117, -2.5224) -> (-5.2877, -2.5224)
  line L10 (-6.0497, -2.5224) -> (-6.0497, -2.7131)
  line L11 (-2.7121, -2.5123) -> (-5.3232, -2.5123)
  line L12 (-5.3232, -2.5123) -> (-5.3232, -3.0406)
  line L13 (-5.3232, -3.0406) -> (-2.7121, -3.0406)
  line L14 (-2.7121, -3.0406) -> (-2.7121, -2.5123)
  line L15 (-2.7477, -3.0304) -> (-5.2877, -3.0304)
  line L16 (-5.2877, -3.0304) -> (-5.2877, -2.5224)
  line L17 (-2.7477, -2.5224) -> (-2.7477, -3.0304)
  line L18 (1.5725, -3.2336) -> (1.5725, -7.9072) projected
  line L19 (1.5725, -7.9072) -> (-0.5611, -7.9072) projected
  line L20 (-0.5611, -7.9072) -> (-0.5611, -3.2336) projected
  line L21 (-0.5611, -3.2336) -> (1.5725, -3.2336) projected
  line L22 (1.7757, -3.0304) -> (-0.7643, -3.0304) projected
  line L23 (-0.7643, -3.0304) -> (-0.7643, -8.1104) projected
  line L24 (-0.7643, -8.1104) -> (1.7757, -8.1104) projected
  line L25 (1.7757, -8.1104) -> (1.7757, -3.0304) projected
  line L26 (-5.2877, -4.8922) -> (-5.2877, -4.3842)
  line L27 (-5.3232, -4.3741) -> (-5.3232, -4.9024)
  line L28 (-2.7477, -4.3842) -> (-2.7477, -4.8922)
  line L29 (-2.7477, -4.8922) -> (-5.2877, -4.8922)
  line L30 (-2.7121, -4.9024) -> (-2.7121, -4.3741)
  line L31 (-5.3232, -4.9024) -> (-2.7121, -4.9024)
  line L32 (-6.7761, -4.3741) -> (-6.7761, -4.9024)
  line L33 (-9.3872, -4.9024) -> (-9.3872, -4.3741)
  line L34 (-6.7761, -4.9024) -> (-9.3872, -4.9024)
  line L35 (-9.3872, -4.3741) -> (-6.7761, -4.3741)
  line L36 (-2.7121, -4.3741) -> (-5.3232, -4.3741)
  line L37 (-5.2877, -6.7541) -> (-5.2877, -6.2461)
  line L38 (-5.3232, -6.2359) -> (-5.3232, -6.7642)
  line L39 (-2.7477, -6.2461) -> (-2.7477, -6.7541)
  line L40 (-2.7477, -6.7541) -> (-5.2877, -6.7541)
  line L41 (-2.7121, -6.7642) -> (-2.7121, -6.2359)
  line L42 (-5.3232, -6.7642) -> (-2.7121, -6.7642)
  line L43 (-6.7761, -6.2359) -> (-6.7761, -6.7642)
  line L44 (-9.3872, -6.7642) -> (-9.3872, -6.2359)
  line L45 (-6.7761, -6.7642) -> (-9.3872, -6.7642)
  line L46 (-9.3872, -6.2359) -> (-6.7761, -6.2359)
  line L47 (-2.7121, -6.2359) -> (-5.3232, -6.2359)
  line L48 (-5.2877, -8.6159) -> (-5.2877, -8.1079)
  line L49 (-5.3232, -8.0977) -> (-5.3232, -8.626)
  line L50 (-2.7477, -8.1079) -> (-2.7477, -8.6159)
  line L51 (-2.7477, -8.6159) -> (-5.2877, -8.6159)
  line L52 (-2.7121, -8.626) -> (-2.7121, -8.0977)
  line L53 (-5.3232, -8.626) -> (-2.7121, -8.626)
  line L54 (-6.7761, -8.0977) -> (-6.7761, -8.626)
  line L55 (-9.3872, -8.626) -> (-9.3872, -8.0977)
  line L56 (-6.7761, -8.626) -> (-9.3872, -8.626)
  line L57 (-9.3872, -8.0977) -> (-6.7761, -8.0977)
  line L58 (-2.7121, -8.0977) -> (-5.3232, -8.0977)
  point P0 (0, 0)
  dimension "d211" = 0.0102
  dimension "d212" = 0.0102
  dimension "d213" = 0.0356
  dimension "d214" = 0.0356
  dimension "d224" = 1.8618
  constraints: 92 end point, 6 symmetric about line, 2 horizontal, 2 parallel, 2 vertical, 1 midpoint, 1 perpendicular, 69 other
  measures "d211" distance between parallel lines of L4 L0
  measures "d212" distance between parallel lines of L5 L2
  measures "d213" distance between parallel lines of L1 L6
  measures "d214" distance between parallel lines of L7 L3
  measures "d224" distance of L15.end L26.start
extrude "Extrusion21" add sketch "Sketch32" along normal blind 0.0127 contours L0 L1 L2 L3 | L14 L13 L12 L11 | L36 L30 L31 L27 | L32 L34 L33 L35 | L47 L41 L42 L38 | L43 L45 L44 L46 | L58 L52 L53 L49 | L54 L56 L55 L57
sketch "Sketch29" plane through (0, 1.524, 0) normal (0, 1, 0) x (1, 0, 0)
  line L0 (-14.1158, -11.874) -> (-13.4623, -11.874) construction
  line L1 (-13.4623, -11.874) -> (-13.4623, -11.8506) construction
  line L2 (-13.4623, -11.8506) -> (-14.1158, -11.8506) construction
  line L3 (-14.1158, -11.8506) -> (-14.1158, -11.874) construction
  line L4 (-11.5961, -11.863) -> (-10.376, -11.863) construction
  line L5 (-10.376, -11.863) -> (-10.376, -12.392) construction
  line L6 (-10.376, -12.392) -> (-11.5961, -12.392) construction
  line L7 (-11.5961, -12.392) -> (-11.5961, -11.863) construction
  line L8 (-9.0608, -11.8448) -> (-7.2144, -11.8448) construction
  line L9 (-7.2144, -11.8448) -> (-7.2144, -12.6339) construction
  line L10 (-7.2144, -12.6339) -> (-9.0608, -12.6339) construction
  line L11 (-9.0608, -12.6339) -> (-9.0608, -11.8448) construction
  line L12 (-6.5821, -11.8706) -> (-5.1754, -11.8706) construction
  line L13 (-5.1754, -11.8706) -> (-5.1754, -12.3976) construction
  line L14 (-5.1754, -12.3976) -> (-6.5821, -12.3976) construction
  line L15 (-6.5821, -12.3976) -> (-6.5821, -11.8706) construction
  line L16 (-3.7618, -11.8575) -> (-2.9068, -11.8575) construction
  line L17 (-2.9068, -11.8575) -> (-2.9068, -12.3762) construction
  line L18 (-2.9068, -12.3762) -> (-3.7618, -12.3762) construction
  line L19 (-3.7618, -12.3762) -> (-3.7618, -11.8575) construction
  line L20 (-1.2411, -11.865) -> (-0.386, -11.865) construction
  line L21 (-0.386, -11.865) -> (-0.386, -12.3944) construction
  line L22 (-0.386, -12.3944) -> (-1.2411, -12.3944) construction
  line L23 (-1.2411, -12.3944) -> (-1.2411, -11.865) construction
  line L24 (1.2577, -11.9005) -> (2.1127, -11.9005) construction
  line L25 (2.1127, -11.9005) -> (2.1127, -12.4085) construction
  line L26 (2.1127, -12.4085) -> (1.2577, -12.4085) construction
  line L27 (1.2577, -12.4085) -> (1.2577, -11.9005) construction
  line L28 (3.8291, -11.8659) -> (4.6841, -11.8659) construction
  line L29 (4.6841, -11.8659) -> (4.6841, -12.3846) construction
  line L30 (4.6841, -12.3846) -> (3.8291, -12.3846) construction
  line L31 (3.8291, -12.3846) -> (3.8291, -11.8659) construction
  line L32 (6.3258, -11.8612) -> (7.1808, -11.8612) construction
  line L33 (7.1808, -11.8612) -> (7.1808, -12.3894) construction
  line L34 (7.1808, -12.3894) -> (6.3258, -12.3894) construction
  line L35 (6.3258, -12.3894) -> (6.3258, -11.8612) construction
  line L36 (8.9419, -11.863) -> (9.7969, -11.863) construction
  line L37 (9.7969, -11.863) -> (9.7969, -13.2074) construction
  line L38 (9.7969, -13.2074) -> (8.9419, -13.2074) construction
  line L39 (8.9419, -13.2074) -> (8.9419, -11.863) construction
  line L40 (11.4181, -11.8604) -> (12.2732, -11.8604) construction
  line L41 (12.2732, -11.8604) -> (12.2732, -12.3914) construction
  line L42 (12.2732, -12.3914) -> (11.4181, -12.3914) construction
  line L43 (11.4181, -12.3914) -> (11.4181, -11.8604) construction
  line L44 (14.0004, -11.862) -> (14.8554, -11.862) construction
  line L45 (14.8554, -11.862) -> (14.8554, -12.3901) construction
  line L46 (14.8554, -12.3901) -> (14.0004, -12.3901) construction
  line L47 (14.0004, -12.3901) -> (14.0004, -11.862) construction
  line L48 (16.2846, -11.8505) -> (17.5209, -11.8505) construction
  line L49 (17.5209, -11.8505) -> (17.5209, -12.3795) construction
  line L50 (17.5209, -12.3795) -> (16.2846, -12.3795) construction
  line L51 (16.2846, -12.3795) -> (16.2846, -11.8505) construction
  line L52 (18.8609, -11.8572) -> (20.0972, -11.8572) construction
  line L53 (20.0972, -11.8572) -> (20.0972, -12.3669) construction
  line L54 (20.0972, -12.3669) -> (18.8609, -12.3669) construction
  line L55 (18.8609, -12.3669) -> (18.8609, -11.8572) construction
  line L56 (21.3858, -11.8471) -> (22.6221, -11.8471) construction
  line L57 (22.6221, -11.8471) -> (22.6221, -12.3658) construction
  line L58 (22.6221, -12.3658) -> (21.3858, -12.3658) construction
  line L59 (21.3858, -12.3658) -> (21.3858, -11.8471) construction
  line L60 (-9.8192, -3.4497) -> (-10.0589, -3.4497) construction
  line L61 (-10.0589, -3.4497) -> (-10.0589, -3.5438) construction
  line L62 (-10.0589, -3.5438) -> (-9.8192, -3.5438) construction
  line L63 (-9.8192, -3.5438) -> (-9.8192, -3.4497) construction
  line L64 (-9.7442, -5.3815) -> (-11.5708, -5.3815) construction
  line L65 (-11.5708, -5.3815) -> (-11.5708, -5.5624) construction
  line L66 (-11.5708, -5.5624) -> (-9.7442, -5.5624) construction
  line L67 (-9.7442, -5.5624) -> (-9.7442, -5.3815) construction
  line L68 (-9.4697, -7.1703) -> (-10.0716, -7.1703) construction
  line L69 (-10.0716, -7.1703) -> (-10.0716, -7.0108) construction
  line L70 (-10.0716, -7.0108) -> (-9.4697, -7.0108) construction
  line L71 (-9.4697, -7.0108) -> (-9.4697, -7.1703) construction
  line L72 (-9.6214, -9.0237) -> (-10.7292, -9.0237) construction
  line L73 (-10.7292, -9.0237) -> (-10.7292, -9.2323) construction
  line L74 (-10.7292, -9.2323) -> (-9.6214, -9.2323) construction
  line L75 (-9.6214, -9.2323) -> (-9.6214, -9.0237) construction
  point P0 (0, 0)
  dimension "d0" = 43.18
  dimension "d1" = 17.78
  constraints: 38 other
body "Solid1"
